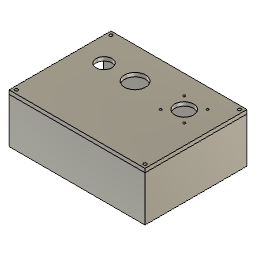
finalProjectBox (Autodesk Fusion 360 design; units mm, degrees)
Autodesk Fusion 360 part; units mm, degrees
sketch "Sketch1" plane through (0, 0, 0) normal (0, 0, 1) x (1, 0, 0)
  line L0 (0, 0) -> (180, 0)
  line L1 (180, 0) -> (180, 135)
  line L2 (180, 135) -> (0, 135)
  line L3 (0, 135) -> (0, 0)
  dimension "d1" = 180
  dimension "d2" = 135
  constraint horizontal L0
  constraint vertical L1
  constraint horizontal L2
  constraint vertical L3
  constraint coincident L0.start L3.end
  measures "d1" distance of L0.start L0.end
  measures "d2" distance of L0.start L2.end
extrude "Extrude1" add sketch "Sketch1" along normal blind 60 makes body 1
sketch "Sketch2" plane through (0, 0, 60) normal (0, 0, 1) x (-1, 0, 0)
  line L0 (0, -135) -> (0, 0)
  line L1 (0, 0) -> (-180, 0)
  line L2 (-180, 0) -> (-180, -135)
  line L3 (-180, -135) -> (0, -135)
  line L4 (-10, -10) -> (-170, -10)
  line L5 (-170, -10) -> (-170, -125)
  line L6 (-170, -125) -> (-10, -125)
  line L7 (-10, -125) -> (0, -125)
  line L8 (-10, -100) -> (0, -100)
  line L9 (0, -100) -> (0, -125)
  line L10 (-10, -100) -> (-10, -10)
  dimension "d5" = 160
  dimension "d6" = 115
  constraint horizontal L4
  constraint vertical L5
  constraint horizontal L6
  constraint coincident L0 L7.end
  constraint perpendicular L0 L7
  constraint coincident L0 L8.end
  constraint perpendicular L0 L8
  constraint perpendicular L4 L10
  measures "d5" distance of L4.start L4.end
  measures "d6" distance of L4.start L6.end
extrude "Extrude2" cut sketch "Sketch2" against normal blind 50 contours L0 L4 L5 L6 L7 L8 L9 L10 bodies 1
sketch "Sketch3" plane through (0, 0, 60) normal (0, 0, 1) x (-1, 0, 0)
  line L0 (-10, -100) -> (0, -100)
  line L1 (0, -100) -> (0, 0)
  line L2 (0, 0) -> (-180, 0)
  line L3 (-180, 0) -> (-180, -135)
  line L4 (-180, -135) -> (0, -135)
  line L5 (0, -135) -> (0, -125)
  line L6 (0, -125) -> (-170, -125)
  line L7 (-170, -125) -> (-170, -10)
  line L8 (-170, -10) -> (-10, -10)
  line L9 (-10, -10) -> (-10, -100)
  circle A0 centre (-5, -5) radius 2
  circle A1 centre (-175, -5) radius 2
  circle A2 centre (-175, -130) radius 2
  circle A3 centre (-5, -130) radius 2
  dimension "d9" = 4
  dimension "d10" = 4
  dimension "d11" = 4
  dimension "d12" = 4
  measures "d9" diameter of A0
  measures "d10" diameter of A1
  measures "d11" diameter of A2
  measures "d12" diameter of A3
extrude "Extrude3" cut sketch "Sketch3" against normal blind 15 contours A0 | A1 | A2 | A3 bodies 1
sketch "Sketch4" plane through (0, 0, 60) normal (0, 0, 1) x (-1, 0, 0)
  circle A0 centre (-5, -5) radius 2
  circle A1 centre (-5, -130) radius 2
  circle A2 centre (-175, -5) radius 2
  circle A3 centre (-175, -130) radius 2
  line L0 (-10, -100) -> (0, -100)
  line L1 (0, -100) -> (0, 0)
  line L2 (0, 0) -> (-180, 0)
  line L3 (-180, 0) -> (-180, -135)
  line L4 (-180, -135) -> (0, -135)
  line L5 (0, -135) -> (0, -125)
  line L6 (0, -125) -> (-170, -125)
  line L7 (-170, -125) -> (-170, -10)
  line L8 (-170, -10) -> (-10, -10)
  line L9 (-10, -10) -> (-10, -100)
  line L10 (0, 0) -> (-180, 0)
  line L11 (-180, 0) -> (-180, -135)
  line L12 (-180, -135) -> (0, -135)
  line L13 (0, -135) -> (0, 0)
  line L14 (-116.82, -115) -> (-116.82, -108.91) construction
  line L15 (-116.82, -108.91) -> (-122.91, -108.91) construction
  circle A4 centre (-122.91, -108.91) radius 1.5
  line L16 (-122.91, -108.91) -> (-153.91, -108.91) construction
  circle A5 centre (-153.91, -108.91) radius 1.5
  line L17 (-153.91, -108.91) -> (-153.91, -77.91) construction
  circle A6 centre (-153.91, -77.91) radius 1.5
  line L18 (-122.91, -108.91) -> (-122.91, -77.91) construction
  circle A7 centre (-122.91, -77.91) radius 1.5
  line L19 (-116.82, -115) -> (-160, -71.82) construction
  line L20 (-116.82, -71.82) -> (-160, -115) construction
  circle A8 centre (-138.41, -93.41) radius 12.5
  line L21 (-138.41, -93.41) -> (-73.41, -93.41) construction
  line L22 (-73.41, -93.41) -> (-32.41, -93.41) construction
  circle A9 centre (-73.41, -93.41) radius 14
  circle A10 centre (-32.41, -93.41) radius 10.5
  dimension "d15" = 43.18
  dimension "d16" = 43.18
  dimension "d17" = 6.09
  dimension "d18" = 6.09
  dimension "d19" = 3
  dimension "d20" = 31
  dimension "d21" = 3
  dimension "d22" = 31
  dimension "d23" = 3
  dimension "d24" = 31
  dimension "d25" = 3
  dimension "d26" = 25
  dimension "d27" = 65
  dimension "d28" = 41
  dimension "d29" = 28
  dimension "d30" = 21
  constraint horizontal L10
  constraint vertical L11
  constraint horizontal L12
  constraint vertical L13
  constraint coincident L3.end L4.start
  constraint coincident L1.end L2.start
  constraint coincident L15.end A4.centre
  constraint parallel L15 L16
  constraint coincident L16.end A5.centre
  constraint perpendicular L16 L17
  constraint coincident L17.end A6.centre
  constraint perpendicular L15 L18
  constraint coincident L18.end A7.centre
  constraint midpoint L20 A8.centre
  constraint coincident A8.centre L21.start
  constraint horizontal L21
  constraint parallel L21 L22
  constraint coincident L21.end L22.start
  constraint coincident L22.end A10.centre
  measures "d15" distance of L20.end L14.start
  measures "d16" distance of L20.end L19.end
  measures "d17" distance of L14.start L14.end
  measures "d18" distance of L14.end L15.end
  measures "d19" diameter of A4
  measures "d20" distance of L15.end L16.end
  measures "d21" diameter of A5
  measures "d22" distance of L16.end L17.end
  measures "d23" diameter of A6
  measures "d24" distance of L15.end L18.end
  measures "d25" diameter of A7
  measures "d26" diameter of A8
  measures "d27" distance of A8.centre L21.end
  measures "d28" distance of L21.end L22.end
  measures "d29" diameter of A9
  measures "d30" diameter of A10
extrude "Extrude4" add sketch "Sketch4" along normal blind 5 separate body makes body 2
named bodies: "MainCasing", "Cover"
